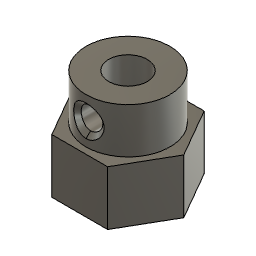
weight (Autodesk Fusion 360 design; units mm, degrees)
Autodesk Fusion 360 part; units mm, degrees
sketch "Esquisse1" plane through (0, 0, 0) normal (0, 1, 0) x (1, 0, 0)
  circle A0 centre (0, 0) radius 4.25
  circle A1 centre (0, 0) radius 9.25
  circle A2 centre (0, 0) radius 5.25
  line L0 (10, 0) -> (5, 8.6603)
  line L1 (5, 8.6603) -> (-5, 8.6603)
  line L2 (-5, 8.6603) -> (-10, 0)
  line L3 (-10, 0) -> (-5, -8.6603)
  line L4 (-5, -8.6603) -> (5, -8.6603)
  line L5 (5, -8.6603) -> (10, 0)
  line L6 (-6.1547, 10.6603) -> (-12.3094, 0)
  line L7 (-12.3094, 0) -> (-6.1547, -10.6603)
  line L8 (-6.1547, -10.6603) -> (6.1547, -10.6603)
  line L9 (6.1547, -10.6603) -> (12.3094, 0)
  line L10 (12.3094, 0) -> (6.1547, 10.6603)
  line L11 (6.1547, 10.6603) -> (-6.1547, 10.6603)
  dimension "d6" = 8.5
  dimension "d7" = 5
  dimension "d19" = 1
  dimension "d25" = 10
  dimension "d26" = 2
  constraint coincident A0.centre A1.centre
  measures "d6" diameter of A0
  measures "d25" distance of L0.start A0.centre
extrude "Extrusion1" add sketch "Esquisse1" along normal blind 10 contours A1 L0 L1 L2 L3 L4 L5 | A1 L0 | A1 L5 | A1 L1 | A1 L4 | A1 L2 | A1 L3 | A2
ref_plane "Plan de construction1" through (0, 6.1987, 9.25) normal (0, 0, 1) x (-1, 0, 0)
sketch "Esquisse2" plane through (0, 6.0312, 9.25) normal (0, 0, 1) x (1, 0, 0)
  line L0 (9.25, 3.9688) -> (-9.25, 3.9688)
  line L1 (9.25, -6.0312) -> (-9.25, -6.0312)
  line L2 (-9.25, 3.9688) -> (9.25, -6.0312) construction
  circle A0 centre (0, -1.0312) radius 2.4
  dimension "d11" = 4.8
  constraint coincident L0.end L2.start
  constraint coincident L1.start L2.end
  constraint midpoint L2 A0.centre
  measures "d11" diameter of A0
extrude "Extrusion2" cut sketch "Esquisse2" against normal blind 9.3
chamfer "Chanfrein1" distance 1 angle 45 2 edges at (2.4, 5, 8.9332) (-2.4, 5, 8.9332)
extrude "Extrusion4" add sketch "Esquisse1" against normal blind 12 contours A0 | A1 L0 L1 L2 L3 L4 L5 | A1 L0 L5 | A1 L0 | A1 L5 | A1 L0 L1 | A1 L4 L5 | A1 L1 | A1 L4 | A1 L1 L2 | A1 L3 L4 | A1 L2 | A1 L3 | A1 L2 L3 | A2 | L6 L7 L8 L9 L10 L11
ref_plane "Plan de construction2" through (0, -2, 0) normal (0, 1, 0) x (1, 0, 0)
sketch "Esquisse3" plane through (0, -2, 0) normal (0, 1, 0) x (1, 0, 0)
  line L0 (10, 0) -> (5, 8.6603)
  line L1 (5, 8.6603) -> (-5, 8.6603)
  line L2 (-5, 8.6603) -> (-10, 0)
  line L3 (-10, 0) -> (-5, -8.6603)
  line L4 (-5, -8.6603) -> (5, -8.6603)
  line L5 (5, -8.6603) -> (10, 0)
extrude "Extrusion5" cut sketch "Esquisse3" against normal blind 8
equation "inner_diam = 8 mm"
equation "insert_len = 4 mm"
equation "margin = 1 mm"
equation "depth = 10 mm"
equation "insert_od = 4.8 mm"
equation "d6 = inner_diam + shaft_tolerance"
equation "d7 = margin + insert_len"
equation "d8 = depth"
equation "d11 = insert_od"
equation "chamfrein = 1 mm"
equation "d13 = -( inner_diam + insert_od * 2 + margin ) / 2"
equation "d15 = chamfrein"
equation "shaft_tolerance = 0.5 mm"
equation "bearing_inner_ring = 1 mm"
equation "spacer_depth = 1 mm"
equation "d19 = bearing_inner_ring"
equation "hex_diam = 20 mm"
equation "hex_depth = 8 mm"
equation "wall = 2 mm"
equation "d25 = hex_diam / 2"
equation "d26 = wall"
equation "d27 = -( wall * 2 + hex_depth )"
equation "d29 = -wall"
equation "d30 = -hex_depth"
